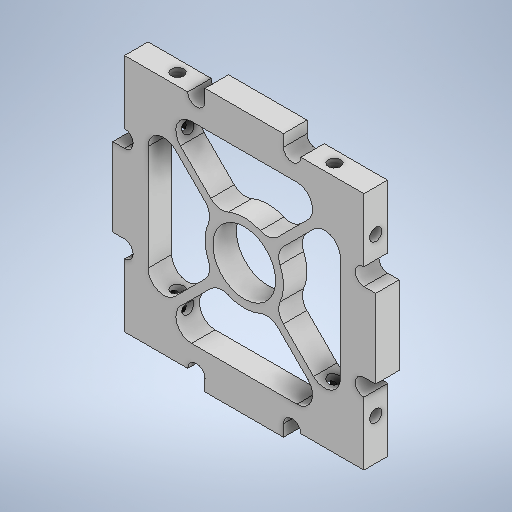
# Autodesk Inventor part: t3kata
Saved by Autodesk Inventor 2025.1 (Build 291241000, 241)
## iProperties
Created: 2024-09-04
Part Number: t3kata
Material: 一般
Document SubType Name: Modeling
Designer: right
Density: 1 g/cm^3
Appearance: 既定
Author: right
Autodesk Inventor part; units mm, degrees
ref_plane "YZ Plane" through (0, 0, 0) normal (1, 0, 0) x (0, 1, 0)
ref_plane "XZ Plane" through (0, 0, 0) normal (0, 1, 0) x (-1, 0, 0)
ref_plane "XY Plane" through (0, 0, 0) normal (0, 0, 1) x (1, 0, 0)
sketch "スケッチ1" plane through (0, 0, 0) normal (0, 0, 1) x (1, 0, 0)
  line L0 (-15.25, -15.25) -> (15.25, -15.25)
  line L1 (15.25, -15.25) -> (15.25, 15.25)
  line L2 (15.25, 15.25) -> (-15.25, 15.25)
  line L3 (-15.25, 15.25) -> (-15.25, -15.25)
  line L4 (-15.25, -15.25) -> (15.25, 15.25) construction
  line L5 (15.25, -15.25) -> (-15.25, 15.25) construction
  line L6 (-5, 15.25) -> (5, 15.25)
  line L7 (5, 15.25) -> (5, 16.75)
  line L8 (5, 16.75) -> (-5, 16.75)
  line L9 (-5, 16.75) -> (-5, 15.25)
  circle A0 centre (0, 0) radius 15.25 construction
  circle A1 centre (-6.1, 15.25) radius 1.1
  line L10 (0, 16.75) -> (0, 15.25) construction
  circle A2 centre (6.1, 15.25) radius 1.1
  circle A3 centre (-15.25, -6.1) radius 1.1
  line L11 (-16.75, 5) -> (-16.75, -5)
  line L12 (-16.75, -5) -> (-15.25, -5)
  line L13 (-15.25, 5) -> (-16.75, 5)
  circle A4 centre (-15.25, 6.1) radius 1.1
  circle A5 centre (6.1, -15.25) radius 1.1
  line L14 (-5, -16.75) -> (5, -16.75)
  line L15 (5, -16.75) -> (5, -15.25)
  line L16 (-5, -15.25) -> (-5, -16.75)
  circle A6 centre (-6.1, -15.25) radius 1.1
  circle A7 centre (15.25, 6.1) radius 1.1
  line L17 (16.75, -5) -> (16.75, 5)
  line L18 (16.75, 5) -> (15.25, 5)
  line L19 (15.25, -5) -> (16.75, -5)
  circle A8 centre (15.25, -6.1) radius 1.1
  point P0 (-16.75, 0)
  point P1 (0, -16.75)
  point P2 (16.75, 0)
  point P3 (-15.25, -7.2)
  point P4 (-7.2, -15.25)
  point P5 (7.2, -15.25)
  point P6 (15.25, -7.2)
  point P7 (15.25, 7.2)
  point P8 (7.2, 15.25)
  point P9 (-7.2, 15.25)
  point P10 (-15.25, 7.2)
  dimension "d3" = 2.2
  dimension "d0" = 30.5
  dimension "d1" = 1.5
  dimension "d2" = 10
  dimension "d6" = 360
  constraints: 40 end point, 4 centre point, 4 midpoint, 4 parallel, 3 horizontal, 3 perpendicular, 2 point on line, 2 vertical alignment, 1 coincident, 1 symmetric about line, 64 other
  measures "d0" distance of L1.end L2.end
  measures "d1" distance between parallel lines of L2 L8
  measures "d2" distance of L7.end L8.end
extrude "押し出し1" add sketch "スケッチ1" along normal blind 3 contours A6 L0 L3 A3 A4 L2 A1 A2 L1 A7 A8 A5 | L0 L15 L14 L16 | L12 L11 L13 L3 | L1 L18 L17 L19 | L9 L8 L7 L2
sketch "スケッチ4" plane through (0, 0, 3) normal (0, 0, 1) x (1, 0, 0)
  line L0 (-12.25, -12.25) -> (12.25, -12.25)
  line L1 (12.25, -12.25) -> (12.25, 12.25)
  line L2 (12.25, 12.25) -> (-12.25, 12.25)
  line L3 (-12.25, 12.25) -> (-12.25, -12.25)
  line L4 (-12.25, -12.25) -> (12.25, 12.25) construction
  line L5 (12.25, -12.25) -> (-12.25, 12.25) construction
  arc A0 (-7.2, 15.25) -> (-5, 15.25) centre (-6.1, 15.25) ccw projected
  arc A1 (-15.25, 5) -> (-15.25, 7.2) centre (-15.25, 6.1) ccw projected
  line L6 (-7.2, 15.25) -> (-15.25, 15.25) projected
  line L7 (-15.25, 15.25) -> (-15.25, 7.2) projected
  circle A2 centre (0, 0) radius 4
  circle A3 centre (0, 0) radius 5
  line L8 (-11.5429, 12.25) -> (12.25, -11.5429)
  line L9 (-12.25, 11.5429) -> (11.5429, -12.25)
  line L10 (0, 12.25) -> (0, 0) construction
  line L11 (11.5429, 12.25) -> (-12.25, -11.5429)
  line L12 (12.25, 11.5429) -> (-11.5429, -12.25)
  point P0 (-6.1, 14.15)
  point P1 (-14.15, 6.1)
  point P2 (-3.1643, -3.8714)
  point P3 (3.1643, -3.8714)
  point P4 (3.8714, 3.1643)
  point P5 (3.8714, -3.1643)
  point P6 (-3.8714, -3.1643)
  point P7 (-3.8714, 3.1643)
  point P8 (3.1643, 3.8714)
  point P9 (-3.1643, 3.8714)
  dimension "d30" = 3
  dimension "d31" = 3
  dimension "d32" = 8
  dimension "d33" = 10
  dimension "d34" = 0.5
  constraints: 22 end point, 6 symmetric about line, 3 midpoint, 3 parallel, 2 centre point, 2 coincident, 2 point on circle, 2 point on line, 1 horizontal, 1 perpendicular, 1 vertical
  measures "d30" distance between parallel lines of L2 L6
  measures "d31" distance between parallel lines of L7 L3
  measures "d32" diameter of A2
  measures "d33" diameter of A3
  measures "d34" distance between parallel lines of L5 L8
extrude "押し出し2" cut sketch "スケッチ4" against normal through all contours L12 A3 L9 L0 | L3 L9 A3 L11 | L12 L9 A2 | A2 L11 L9 L12 | A2 L9 L11 | L8 A3 L12 L1 | L9 L12 L8 A2 | L9 L11 L8 L12 | L2 L11 A3 L8 | A2 L8 L11 L9 | L8 L12 A2 | L8 L11 A2 L12 | A2 L11 L8
fillet "フィレット1" radius 2 16 edges at (-12.25, 11.5429, 1.5) (-11.5429, 12.25, 1.5) (12.25, 11.5429, 1.5) (11.5429, 12.25, 1.5) (11.5429, -12.25, 1.5) (12.25, -11.5429, 1.5) (-11.5429, -12.25, 1.5) (-12.25, -11.5429, 1.5) (-3.1643, -3.8714, 1.5) (3.1643, -3.8714, 1.5) (3.8714, -3.1643, 1.5) (3.8714, 3.1643, 1.5) (3.1643, 3.8714, 1.5) (-3.1643, 3.8714, 1.5) (-3.8714, 3.1643, 1.5) (-3.8714, -3.1643, 1.5)
sketch "スケッチ2" plane through (-15.25, 7.2, 0) normal (-1, 0, 0) x (0, 0, 1)
  line L0 (0, -2.2) -> (3, -2.2) projected
  line L1 (0, -12.2) -> (3, -12.2) projected
  point P0 (0, -7.2)
  point P1 (1.5, 2.8)
  point P2 (1.5, -17.2)
  point P3 (1.5, -2.2)
  point P4 (1.5, -12.2)
  point P5 (1.5, -2.2)
  point P6 (1.5, -12.2)
  dimension "d10" = 5
  dimension "d11" = 5
  constraints: 4 midpoint, 2 vertical alignment
  measures "d10" distance of point (1.5, 2.8) point (1.5, -2.2)
  measures "d11" distance of point (1.5, -17.2) point (1.5, -12.2)
hole "穴1" at (-15.25, 10, 1.5) at (-15.25, -10, 1.5) direction (1, 0, 0) diameter 1.567 end through all thread size "M2x0.4" class "6H" standard "ISO Metric profile"
sketch "スケッチ3" plane through (-15.25, 15.25, 0) normal (0, 1, 0) x (1, 0, 0)
  line L0 (10.25, 0) -> (10.25, -3) projected
  line L1 (20.25, 0) -> (20.25, -3) projected
  point P0 (15.25, 0)
  point P1 (5.25, -1.5)
  point P2 (25.25, -1.5)
  point P3 (10.25, -1.5)
  point P4 (20.25, -1.5)
  point P5 (10.25, -1.5)
  point P6 (20.25, -1.5)
  dimension "d19" = 5
  dimension "d20" = 5
  constraints: 4 midpoint, 2 horizontal alignment
  measures "d19" distance of point (10.25, -1.5) point (5.25, -1.5)
  measures "d20" distance of point (20.25, -1.5) point (25.25, -1.5)
hole "穴2" at (-10, 15.25, 1.5) at (10, 15.25, 1.5) direction (0, -1, 0) diameter 1.567 end through all thread size "M2x0.4" class "6H" standard "ISO Metric profile"
equation "\"d31\" = d30"
equation "\"d11\" = d10"
equation "\"d20\" = d19"
